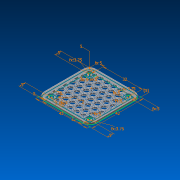
# Autodesk Inventor part: 40mm fan grill hex
Saved by Autodesk Inventor 2015 (Build 190159000, 159)
## iProperties
Created: 2017-03-15
Part Number: 40mm fan grill hex
Material: Generic
Document SubType Name: Modeling
Designer: ZigZagJoe
Density: 1 g/cm^3
Appearance: Default
Author: ZigZagJoe
Autodesk Inventor part; units mm, degrees
ref_plane "YZ Plane" through (0, 0, 0) normal (1, 0, 0) x (0, 1, 0)
ref_plane "XZ Plane" through (0, 0, 0) normal (0, 1, 0) x (-1, 0, 0)
ref_plane "XY Plane" through (0, 0, 0) normal (0, 0, 1) x (1, 0, 0)
sketch "Sketch1" plane through (0, 0, 0) normal (0, 0, 1) x (1, 0, 0)
  line L0 (-12.0516, 15.6269) -> (19.9484, 15.6269)
  line L1 (24.9484, 10.6269) -> (24.9484, -21.3731)
  line L2 (19.9484, -26.3731) -> (-12.0516, -26.3731)
  line L3 (-17.0516, -21.3731) -> (-17.0516, 10.6269)
  circle A0 centre (-12.0516, -21.3731) radius 1.875
  circle A1 centre (-12.0516, 10.6269) radius 1.875
  circle A2 centre (19.9484, 10.6269) radius 1.875
  circle A3 centre (19.9484, -21.3731) radius 1.875
  arc A4 (-12.0516, 15.6269) -> (-17.0516, 10.6269) centre (-12.0516, 10.6269) ccw
  arc A5 (24.9484, 10.6269) -> (19.9484, 15.6269) centre (19.9484, 10.6269) ccw
  arc A6 (19.9484, -26.3731) -> (24.9484, -21.3731) centre (19.9484, -21.3731) ccw
  arc A7 (-17.0516, -21.3731) -> (-12.0516, -26.3731) centre (-12.0516, -21.3731) ccw
  line L4 (-14.0516, 12.6269) -> (-9.0516, 12.6269)
  line L5 (-9.0516, 12.6269) -> (-9.0516, 9.6269)
  line L6 (-11.0516, 7.6269) -> (-14.0516, 7.6269)
  line L7 (-14.0516, 7.6269) -> (-14.0516, 12.6269)
  line L8 (21.9484, 12.6269) -> (16.9484, 12.6269)
  line L9 (16.9484, 12.6269) -> (16.9484, 9.6269)
  line L10 (18.9484, 7.6269) -> (21.9484, 7.6269)
  line L11 (21.9484, 7.6269) -> (21.9484, 12.6269)
  line L12 (21.9484, -23.3731) -> (16.9484, -23.3731)
  line L13 (16.9484, -23.3731) -> (16.9484, -20.3731)
  line L14 (18.9484, -18.3731) -> (21.9484, -18.3731)
  line L15 (21.9484, -18.3731) -> (21.9484, -23.3731)
  line L16 (-14.0516, -23.3731) -> (-9.0516, -23.3731)
  line L17 (-9.0516, -23.3731) -> (-9.0516, -20.3731)
  line L18 (-11.0516, -18.3731) -> (-14.0516, -18.3731)
  line L19 (-14.0516, -18.3731) -> (-14.0516, -23.3731)
  line L20 (-9.0516, 12.6269) -> (16.9484, 12.6269)
  line L21 (21.9484, -18.3731) -> (21.9484, 7.6269)
  line L22 (16.9484, -23.3731) -> (-9.0516, -23.3731)
  line L23 (-14.0516, -18.3731) -> (-14.0516, 7.6269)
  arc A8 (-9.0516, -20.3731) -> (-11.0516, -18.3731) centre (-11.0516, -20.3731) ccw
  arc A9 (18.9484, -18.3731) -> (16.9484, -20.3731) centre (18.9484, -20.3731) ccw
  arc A10 (16.9484, 9.6269) -> (18.9484, 7.6269) centre (18.9484, 9.6269) ccw
  arc A11 (-11.0516, 7.6269) -> (-9.0516, 9.6269) centre (-11.0516, 9.6269) ccw
  point P0 (0, 0)
  point P1 (24.9484, -26.3731)
  point P2 (24.9484, 15.6269)
  point P3 (-17.0516, -26.3731)
  point P4 (-9.0516, 7.6269)
  point P5 (16.9484, 7.6269)
  point P6 (16.9484, -18.3731)
  point P7 (-9.0516, -18.3731)
  dimension "d0" = 42
  dimension "d1" = 42
  dimension "d2" = 3.75
  dimension "d3" = 3.75
  dimension "d4" = 3.75
  dimension "d5" = 3.75
  dimension "d7" = 32
  dimension "d8" = 32
  dimension "d9" = 5
  dimension "d11" = 5
  dimension "d12" = 5
  dimension "d13" = 5
  dimension "d14" = 5
  dimension "d15" = 5
  dimension "d18" = 5
  dimension "d19" = 5
  dimension "d84" = 5
  dimension "d85" = 5
  dimension "d86" = 5
  dimension "d87" = 5
  dimension "d88" = 5
  dimension "d89" = 5
  dimension "d90" = 5
  dimension "d91" = 2
  dimension "d94" = 2
  dimension "d95" = 2
  dimension "d97" = 2
  dimension "d98" = 2
  constraints: 48 end point, 16 point on circle, 16 tangent, 15 point on line, 12 centre point, 10 parallel, 7 horizontal, 7 perpendicular, 6 equal radius
  measures "d0" distance of point (24.948, -26.373) point (-17.052, -26.373)
  measures "d1" distance of point (24.948, 15.627) point (24.948, -26.373)
  measures "d2" diameter of A0
  measures "d3" diameter of A1
  measures "d4" diameter of A2
  measures "d5" diameter of A3
  measures "d7" distance of A2.centre A1.centre
  measures "d8" distance of A3.centre A0.centre
  measures "d9" distance from line of L3 A1.centre
  measures "d11" distance from line of L0 A1.centre
  measures "d12" distance from line of L0 A2.centre
  measures "d13" distance from line of L1 A2.centre
  measures "d14" distance from line of L2 A0.centre
  measures "d15" distance from line of L3 A0.centre
  measures "d18" distance from line of L2 A3.centre
  measures "d19" radius of A4
  measures "d84" distance of point (-9.052, -18.373) L18.end
  measures "d85" distance of L16.end point (-9.052, -18.373)
  measures "d86" distance of point (16.948, -18.373) L14.end
  measures "d87" distance of point (16.948, 7.627) L10.end
  measures "d88" distance of L8.end point (16.948, 7.627)
  measures "d89" distance of L4.end point (-9.052, 7.627)
  measures "d90" distance of point (-9.052, 7.627) L6.end
  measures "d91" horizontal distance of L4.start A1.centre
  measures "d94" distance from line of L16 A0.centre
  measures "d95" distance from line of L15 A6.centre
  measures "d97" distance from line of L8 A5.centre
  measures "d98" radius of A8
extrude "Extrusion1" add sketch "Sketch1" along normal blind 1.5 contours L0 A5 L1 A6 L2 A7 L3 A4 | A0 | A1 | A2 | A3 | L4 L5 A11 L6 L7 | L20 L9 A10 L10 L21 L14 A9 L13 L22 L17 A8 L18 L23 L6 A11 L5 | L8 L11 L10 A10 L9 | L18 A8 L17 L16 L19 | L15 L12 L13 A9 L14
sketch "Sketch2" plane through (0, 0, 1.5) normal (0, 0, 1) x (1, 0, 0)
  line L0 (-17.8016, 19.2353) -> (-19.8016, 18.0806)
  line L1 (-19.8016, 18.0806) -> (-21.8016, 19.2353)
  line L2 (-21.8016, 19.2353) -> (-21.8016, 21.5447)
  line L3 (-21.8016, 21.5447) -> (-19.8016, 22.6994)
  line L4 (-19.8016, 22.6994) -> (-17.8016, 21.5447)
  line L5 (-17.8016, 21.5447) -> (-17.8016, 19.2353)
  line L6 (-17.0516, 17.9363) -> (-15.0516, 16.7816)
  line L7 (-15.0516, 16.7816) -> (-15.0516, 14.4722)
  line L8 (-15.0516, 14.4722) -> (-17.0516, 13.3175)
  line L9 (-17.0516, 13.3175) -> (-19.0516, 14.4722)
  line L10 (-19.0516, 14.4722) -> (-19.0516, 16.7816)
  line L11 (-19.0516, 16.7816) -> (-17.0516, 17.9363)
  line L12 (-17.0516, 10.6269) -> (-17.0516, -21.3731) projected
  line L13 (19.9484, 15.6269) -> (-12.0516, 15.6269) projected
  line L14 (-20.5516, 16.7816) -> (-20.5516, 14.4722)
  line L15 (-20.5516, 14.4722) -> (-22.5516, 13.3175)
  line L16 (-22.5516, 13.3175) -> (-24.5516, 14.4722)
  line L17 (-24.5516, 14.4722) -> (-24.5516, 16.7816)
  line L18 (-24.5516, 16.7816) -> (-22.5516, 17.9363)
  line L19 (-22.5516, 17.9363) -> (-20.5516, 16.7816)
  line L20 (-19.8016, 13.1732) -> (-17.8016, 12.0185)
  line L21 (-17.8016, 12.0185) -> (-17.8016, 9.7091)
  line L22 (-17.8016, 9.7091) -> (-19.8016, 8.5544)
  line L23 (-19.8016, 8.5544) -> (-21.8016, 9.7091)
  line L24 (-21.8016, 9.7091) -> (-21.8016, 12.0185)
  line L25 (-21.8016, 12.0185) -> (-19.8016, 13.1732)
  line L26 (-16.3016, 12.0185) -> (-14.3016, 13.1732)
  line L27 (-14.3016, 13.1732) -> (-12.3016, 12.0185)
  line L28 (-12.3016, 12.0185) -> (-12.3016, 9.7091)
  line L29 (-12.3016, 9.7091) -> (-14.3016, 8.5544)
  line L30 (-14.3016, 8.5544) -> (-16.3016, 9.7091)
  line L31 (-16.3016, 9.7091) -> (-16.3016, 12.0185)
  line L32 (-13.5516, 14.4722) -> (-13.5516, 16.7816)
  line L33 (-13.5516, 16.7816) -> (-11.5516, 17.9363)
  line L34 (-11.5516, 17.9363) -> (-9.5516, 16.7816)
  line L35 (-9.5516, 16.7816) -> (-9.5516, 14.4722)
  line L36 (-9.5516, 14.4722) -> (-11.5516, 13.3175)
  line L37 (-11.5516, 13.3175) -> (-13.5516, 14.4722)
  line L38 (-14.3016, 18.0806) -> (-16.3016, 19.2353)
  line L39 (-16.3016, 19.2353) -> (-16.3016, 21.5447)
  line L40 (-16.3016, 21.5447) -> (-14.3016, 22.6994)
  line L41 (-14.3016, 22.6994) -> (-12.3016, 21.5447)
  line L42 (-12.3016, 21.5447) -> (-12.3016, 19.2353)
  line L43 (-12.3016, 19.2353) -> (-14.3016, 18.0806)
  point P0 (0, 0)
  point P1 (-19.8016, 20.39)
  point P2 (-17.0516, 15.6269)
  dimension "d54" = 1.5
  dimension "d55" = 0.75
  dimension "d56" = 4
  dimension "d57" = 4
  dimension "d58" = 1.5
  dimension "d59" = 0
  dimension "d66" = 360
  constraints: 84 end point, 99 other
  measures "d54" distance of L10.end L0.end
  measures "d55" horizontal distance of L10.end L0.end
  measures "d56" distance between parallel lines of L8 L11
  measures "d57" distance between parallel lines of L0 L3
  measures "d58" distance of L0.start L6.start
  measures "d59" angle of L12 L2
extrude "Extrusion4" cut sketch "Sketch2" against normal blind 10
pattern_linear "Rectangular Pattern1" count 5 spacing 11 along (1, 0, 0) count 5 spacing 9.5 along (0, -1, 0) of "Extrusion4"
sketch "Sketch3" plane through (0, 0, 1.5) normal (0, 0, 1) x (1, 0, 0)
  point P0 (0, 0)
extrude "Extrusion5" add sketch "Sketch1" along normal blind 1.5 contours L0 A5 L1 A6 L2 A7 L3 A4 | A0 | A1 | A2 | A3 | L4 L5 A11 L6 L7 | L8 L11 L10 A10 L9 | L18 A8 L17 L16 L19 | L15 L12 L13 A9 L14
extrude "Extrusion6" cut sketch "Sketch1" along normal blind 2 contours A0 | A1 | A2 | A3
equation "\"d3\" = d2"
equation "\"d4\" = d2"
equation "\"d5\" = d2"
equation "\"d9\" = d13"
equation "\"d12\" = d11"
equation "\"d85\" = d84"
equation "\"d86\" = d84"
equation "\"d87\" = d84"
equation "\"d88\" = d84"
equation "\"d89\" = d84"
equation "\"d90\" = d84"
equation "\"d55\" = 0.5 * d54"
equation "\"d57\" = d56"
equation "\"d58\" = d54"
body "Solid1"
